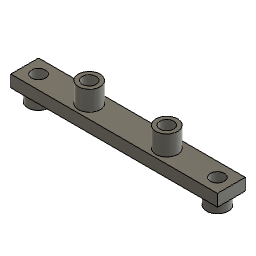
Troodon_2_LIS3DH_Mount_v1 (Autodesk Fusion 360 design; units mm, degrees)
Autodesk Fusion 360 part; units mm, degrees
note: some values were not read from the file. Set by a fixed rule: which sketch regions a step uses.
sketch "Sketch1" plane through (0, 0, 0) normal (0, 1, 0) x (1, 0, 0)
  line L0 (0, 0) -> (22.5, 0)
  line L1 (0, 0) -> (-22.5, 0)
  circle A0 centre (22.5, 0) radius 1.75
  circle A1 centre (-22.5, 0) radius 1.75
  circle A2 centre (-22.5, 0) radius 2.75
  circle A3 centre (22.5, 0) radius 2.75
  line L2 (-26, 3.5) -> (26, 3.5)
  line L3 (26, 3.5) -> (26, -3.5)
  line L4 (26, -3.5) -> (-26, -3.5)
  line L5 (-26, -3.5) -> (-26, 3.5)
  dimension "d1" = 22.5
  dimension "d2" = 22.5
  dimension "d3" = 3.5
  dimension "d4" = 3.5
  dimension "d5" = 5.5
  dimension "d6" = 5.5
  dimension "d7" = 3.5
  dimension "d8" = 3.5
  dimension "d9" = 3.5
  dimension "d10" = 3.5
  constraint coincident L0.start L1.start
  constraint horizontal L0
  constraint parallel L0 L1
  constraint coincident L0.end A0.centre
  constraint coincident L1.end A1.centre
  constraint concentric A1 A2
  constraint concentric A0 A3
  constraint horizontal L2
  constraint vertical L3
  constraint horizontal L4
  constraint vertical L5
  measures "d1" distance of L0.start L0.end
  measures "d2" distance of L0.start L1.end
  measures "d3" diameter of A0
  measures "d4" diameter of A1
  measures "d5" diameter of A2
  measures "d6" diameter of A3
  measures "d7" distance of L0.start L4
  measures "d8" distance of L0.start L2
  measures "d9" distance of L1.end L5
  measures "d10" distance of L0.end L3
extrude "Extrude1" add sketch "Sketch1" along normal blind 3 contours A0 | A1 | A2 | A3 | L2 L3 L4 L5
extrude "Extrude2" add sketch "Sketch1" against normal blind 3 contours A2 | A3
extrude "Extrude3" cut sketch "Sketch1" along normal through all contours A0 | A1
sketch "Sketch2" plane through (0, 3, 0) normal (0, 1, 0) x (-1, 0, 0)
  circle A0 centre (22.5, 0) radius 1.75
  circle A1 centre (-22.5, 0) radius 1.75
  line L0 (26, 3.5) -> (-26, 3.5)
  line L1 (-26, 3.5) -> (-26, -3.5)
  line L2 (-26, -3.5) -> (26, -3.5)
  line L3 (26, -3.5) -> (26, 3.5)
  circle A2 centre (9.75, 0) radius 2.75
  circle A3 centre (-9.75, 0) radius 2.75
  line L4 (9.75, 0) -> (-9.75, 0) construction
  circle A4 centre (9.75, 0) radius 1.75
  circle A5 centre (-9.75, 0) radius 1.75
  dimension "d16" = 9.75
  dimension "d17" = 9.75
  dimension "d18" = 5.5
  dimension "d19" = 5.5
  dimension "d20" = 3.5
  dimension "d21" = 3.5
  constraint coincident A2.centre L4.start
  constraint coincident A3.centre L4.end
  constraint horizontal L4
  constraint concentric A2 A4
  measures "d16" distance of origin A2.centre
  measures "d17" distance of origin A3.centre
  measures "d18" diameter of A2
  measures "d19" diameter of A3
  measures "d20" diameter of A4
  measures "d21" diameter of A5
extrude "Extrude4" add sketch "Sketch2" along normal blind 5 contours A2 | A3
sketch "Sketch3" plane through (0, 0, 0) normal (0, 1, 0) x (1, 0, 0)
  circle A0 centre (9.75, 0.0234) radius 2.75
  circle A1 centre (-9.75, 0.0234) radius 2.75
  line L0 (7, 0.0234) -> (8.375, -2.3582)
  line L1 (8.375, -2.3582) -> (11.125, -2.3582)
  line L2 (11.125, -2.3582) -> (12.5, 0.0234)
  line L3 (12.5, 0.0234) -> (11.125, 2.4049)
  line L4 (11.125, 2.4049) -> (8.375, 2.4049)
  line L5 (8.375, 2.4049) -> (7, 0.0234)
  line L6 (-12.5, 0.0234) -> (-11.125, -2.3582)
  line L7 (-11.125, -2.3582) -> (-8.375, -2.3582)
  line L8 (-8.375, -2.3582) -> (-7, 0.0234)
  line L9 (-7, 0.0234) -> (-8.375, 2.4049)
  line L10 (-8.375, 2.4049) -> (-11.125, 2.4049)
  line L11 (-11.125, 2.4049) -> (-12.5, 0.0234)
  point P0 (9.75, 0.0234)
  point P1 (-9.75, 0.0234)
  dimension "d24" = 5.5
  dimension "d25" = 5.5
  dimension "d26" = 9.75
  dimension "d27" = 9.75
  constraint coincident P0 A0.centre
  constraint coincident A0 L0.start
  constraint coincident P1 A1.centre
  constraint coincident A1 L6.start
  measures "d24" diameter of A0
  measures "d25" diameter of A1
  measures "d26" horizontal distance of origin A0.centre
  measures "d27" horizontal distance of origin P1
extrude "Extrude5" cut sketch "Sketch3" along normal blind 2 contours L0 L1 L2 L3 L4 L5 | L6 L7 L8 L9 L10 L11
extrude "Extrude6" cut 2 faces at (-10.0464, 3, -0.5687) (9.3674, 3, -0.5817) along direction (0, -1, 0) through all
equation "d1 = ( 45 / 2 ) * 1 mm"
equation "d2 = ( 45 / 2 ) * 1 mm"
equation "d16 = ( 19.5 / 2 ) * 1 mm"
equation "d17 = ( 19.5 / 2 ) * 1 mm"
equation "d26 = ( 19.5 / 2 ) * 1 mm"
equation "d27 = ( 19.5 / 2 ) * 1 mm"
